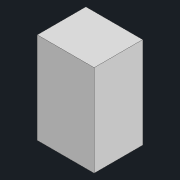
# Autodesk Inventor part: TEaching
Saved by Autodesk Inventor 2022 (Build 260153000, 153)
## iProperties
Created: 2021-09-17
Part Number: TEaching
Material: Generic
Document SubType Name: Modeling
Designer: divid
Density: 1 g/cm^3
Appearance: Default
Author: divid
Autodesk Inventor part; units mm, degrees
ref_plane "YZ Plane" through (0, 0, 0) normal (1, 0, 0) x (0, 1, 0)
ref_plane "XZ Plane" through (0, 0, 0) normal (0, 1, 0) x (-1, 0, 0)
ref_plane "XY Plane" through (0, 0, 0) normal (0, 0, 1) x (1, 0, 0)
sketch "Sketch1" plane through (0, 0, 0) normal (0, 1, 0) x (-1, 0, 0)
  line L0 (0, 0) -> (-15.7882, 0)
  line L1 (-15.7882, 0) -> (-15.7882, 13.4862)
  line L2 (-15.7882, 13.4862) -> (0, 13.4862)
  line L3 (0, 13.4862) -> (0, 0)
  constraints: 8 end point, 2 parallel, 1 horizontal, 1 perpendicular
extrude "Extrusion1" add sketch "Sketch1" along normal blind 25.4
body "Solid1"
